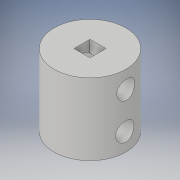
# Autodesk Inventor part: Part2
Saved by Autodesk Inventor 2018 (Build 220112000, 112)
## iProperties
Created: 2018-03-06
Part Number: Part2
Material: Generic
Document SubType Name: Modeling
Designer: prakh
Density: 1 g/cm^3
Appearance: Default
Author: prakh
Autodesk Inventor part; units mm, degrees
ref_plane "YZ Plane" through (0, 0, 0) normal (1, 0, 0) x (0, 1, 0)
ref_plane "XZ Plane" through (0, 0, 0) normal (0, 1, 0) x (-1, 0, 0)
ref_plane "XY Plane" through (0, 0, 0) normal (0, 0, 1) x (1, 0, 0)
sketch "Sketch1" plane through (0, 0, 0) normal (0, 1, 0) x (-1, 0, 0)
  line L0 (2.1273, 2.1273) -> (-2.1273, 2.1273)
  line L1 (-2.1273, 2.1273) -> (-2.1273, -2.1273)
  line L2 (-2.1273, -2.1273) -> (2.1273, -2.1273)
  line L3 (2.1273, -2.1273) -> (2.1273, 2.1273)
  circle A0 centre (0, 0) radius 9.525
  point P0 (2.1273, 0)
  point P1 (0, -2.1272)
  dimension "d0" = 4.2545
  dimension "d1" = 19.05
  constraints: 8 end point, 2 midpoint, 2 parallel, 2 perpendicular, 1 centre point, 1 coincident, 1 horizontal, 1 horizontal alignment, 1 vertical alignment
  measures "d0" distance of L2.end L0.start
  measures "d1" diameter of A0
extrude "Extrusion1" add sketch "Sketch1" along normal blind 9.525
sketch "Sketch2" plane through (0, 0, 0) normal (0, -1, 0) x (1, 0, 0)
  line L0 (-4.7625, 2.7496) -> (0, 5.4993)
  line L1 (0, 5.4993) -> (4.7625, 2.7496)
  line L2 (4.7625, 2.7496) -> (4.7625, -2.7496)
  line L3 (4.7625, -2.7496) -> (0, -5.4993)
  line L4 (0, -5.4993) -> (-4.7625, -2.7496)
  line L5 (-4.7625, -2.7496) -> (-4.7625, 2.7496)
  circle A0 centre (0, 0) radius 9.525 projected
  dimension "d4" = 9.525
  constraints: 12 end point, 1 coincident, 1 vertical, 13 other
  measures "d4" distance between parallel lines of L2 L5
extrude "Extrusion2" add sketch "Sketch2" along normal blind 9.525
sketch "Sketch3" plane through (0, 0, 0) normal (1, 0, 0) x (0, 1, 0)
  circle A0 centre (-4.7625, 0) radius 2.4447
  circle A1 centre (4.7625, -0.254) radius 2.4447
  line L0 (0, 2.1273) -> (9.525, 2.1273) projected
  line L1 (0, 2.7496) -> (-9.525, 2.7496) projected
  point P0 (0, 0)
  point P1 (-4.7625, 2.7496)
  point P2 (4.7625, 2.1273)
  dimension "d7" = 4.8895
  dimension "d8" = 4.8895
  constraints: 2 centre point, 2 midpoint, 2 vertical alignment
  measures "d7" diameter of A0
  measures "d8" diameter of A1
extrude "Extrusion3" cut sketch "Sketch3" along normal mid plane 19.05
body "Solid1"
